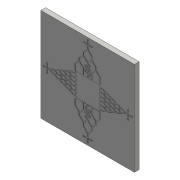
# Autodesk Inventor part: Tree+Mixer
Saved by Autodesk Inventor 2016 (Build 200138000, 138)
## iProperties
Created: 2018-10-05
Part Number: Tree+Mixer
Material: Genérico
Document SubType Name: Modeling
Designer: Joseahpacho
Density: 1 g/cm^3
Appearance: Valor por defecto
Author: Joseahpacho
Autodesk Inventor part; units mm, degrees
ref_plane "YZ Plane" through (0, 0, 0) normal (1, 0, 0) x (0, 1, 0)
ref_plane "XZ Plane" through (0, 0, 0) normal (0, 1, 0) x (-1, 0, 0)
ref_plane "XY Plane" through (0, 0, 0) normal (0, 0, 1) x (1, 0, 0)
sketch "Boceto1" plane through (0, 0, 0) normal (0, 1, 0) x (-1, 0, 0)
  line L0 (29.6771, 58.45) -> (33.6771, 60.45)
  line L1 (23.4615, 55.55) -> (24.4631, 55.55)
  line L2 (24.4631, 55.55) -> (27.5631, 54)
  line L3 (24.4631, 52.45) -> (27.5631, 54)
  line L4 (25.5755, 56) -> (28.6755, 57.55)
  line L5 (25.5755, 56) -> (28.6755, 54.45)
  line L6 (25.5755, 52) -> (28.6755, 50.45)
  line L7 (23.4615, 52.45) -> (24.4631, 52.45)
  line L8 (23.4615, 52.45) -> (24.4631, 52.45)
  line L9 (24.4631, 52.45) -> (23.4615, 52.45)
  line L10 (25.3631, 48) -> (28.4631, 49.55)
  line L11 (24.4631, 51.55) -> (27.4568, 50.0531)
  line L12 (23.4615, 51.55) -> (24.4631, 51.55)
  line L13 (23.4615, 51.55) -> (24.4631, 51.55)
  line L14 (24.2506, 48.45) -> (27.4568, 50.0531)
  line L15 (23.4615, 48.45) -> (24.2506, 48.45)
  line L16 (24.2506, 48.45) -> (23.4615, 48.45)
  line L17 (23.4615, 48.45) -> (24.2506, 48.45)
  line L18 (33.8896, 56.45) -> (35.8375, 56.45)
  line L19 (29.4647, 54.45) -> (32.6709, 56.0531)
  line L20 (33.6771, 52.45) -> (36.0499, 52.45)
  line L21 (33.6771, 51.55) -> (36.0499, 51.55)
  line L22 (29.4647, 53.55) -> (32.5647, 52)
  line L23 (29.4647, 50.45) -> (32.5647, 52)
  line L24 (29.4647, 54.45) -> (28.6755, 54.45)
  line L25 (28.6755, 54.45) -> (29.4647, 54.45)
  line L26 (29.4647, 53.55) -> (28.6755, 53.55)
  line L27 (28.6755, 53.55) -> (29.4647, 53.55)
  line L28 (28.4631, 49.55) -> (29.4647, 49.55)
  line L29 (28.4631, 49.55) -> (29.4647, 49.55)
  line L30 (29.4647, 49.55) -> (28.4631, 49.55)
  line L31 (29.4647, 50.45) -> (28.6755, 50.45)
  line L32 (28.6755, 50.45) -> (29.4647, 50.45)
  line L33 (28.6755, 50.45) -> (29.4647, 50.45)
  line L34 (28.6755, 54.45) -> (29.4647, 54.45)
  line L35 (29.4647, 49.55) -> (32.4585, 48.0531)
  line L36 (30.5771, 50) -> (33.6771, 48.45)
  line L37 (30.5771, 50) -> (33.6771, 51.55)
  line L38 (33.4647, 47.55) -> (36.0499, 47.55)
  line L39 (33.6771, 48.45) -> (36.0499, 48.45)
  line L40 (30.5771, 54) -> (33.6771, 52.45)
  line L41 (30.5771, 54) -> (33.6771, 55.55)
  line L42 (33.6771, 52.45) -> (35.8375, 52.45)
  line L43 (33.6771, 55.55) -> (35.8375, 55.55)
  line L44 (33.6771, 55.55) -> (36.0499, 55.55)
  line L45 (33.8896, 56.45) -> (36.0499, 56.45)
  line L46 (28.6755, 53.55) -> (29.4647, 53.55)
  line L47 (29.2522, 46.45) -> (28.4631, 46.45)
  line L48 (28.4631, 46.45) -> (29.2522, 46.45)
  line L49 (33.4647, 47.55) -> (35.625, 47.55)
  line L50 (28.4631, 46.45) -> (29.2522, 46.45)
  line L51 (28.2506, 45.55) -> (29.2522, 45.55)
  line L52 (28.2506, 45.55) -> (29.2522, 45.55)
  line L53 (33.4647, 44.45) -> (35.625, 44.45)
  line L54 (33.4647, 44.45) -> (36.0499, 44.45)
  line L55 (29.2522, 45.55) -> (32.246, 44.0531)
  line L56 (29.0398, 42.45) -> (32.246, 44.0531)
  line L57 (30.1522, 42) -> (33.2522, 43.55)
  line L58 (33.2522, 40.45) -> (36.0499, 40.45)
  line L59 (33.0398, 39.55) -> (36.0499, 39.55)
  line L60 (30.1522, 42) -> (33.2522, 40.45)
  line L61 (28.2506, 42.45) -> (29.0398, 42.45)
  line L62 (29.0398, 42.45) -> (28.2506, 42.45)
  line L63 (28.0382, 41.55) -> (29.0398, 41.55)
  line L64 (29.0398, 41.55) -> (28.0382, 41.55)
  line L65 (25.1506, 44) -> (28.2506, 42.45)
  line L66 (24.2506, 47.55) -> (27.2444, 46.0531)
  line L67 (15.1474, 48) -> (18.2474, 46.45)
  line L68 (19.0366, 45.55) -> (18.035, 45.55)
  line L69 (20.3615, 54) -> (23.4615, 55.55)
  line L70 (20.3615, 54) -> (23.4615, 52.45)
  line L71 (19.249, 54.45) -> (23.249, 56.45)
  line L72 (19.0366, 46.45) -> (22.2428, 48.0531)
  line L73 (19.249, 53.55) -> (22.349, 52)
  line L74 (19.249, 54.45) -> (18.2474, 54.45)
  line L75 (19.249, 53.55) -> (18.2474, 53.55)
  line L76 (18.2474, 53.55) -> (19.249, 53.55)
  line L77 (18.035, 54.45) -> (19.249, 54.45)
  line L78 (19.249, 50.45) -> (22.349, 52)
  line L79 (24.4631, 55.55) -> (23.4615, 55.55)
  line L80 (20.3615, 50) -> (23.4615, 51.55)
  line L81 (20.3615, 50) -> (23.4615, 48.45)
  line L82 (20.149, 46) -> (23.249, 44.45)
  line L83 (20.149, 46) -> (23.249, 47.55)
  line L84 (19.249, 49.55) -> (22.2428, 48.0531)
  line L85 (19.249, 50.45) -> (18.2474, 50.45)
  line L86 (19.249, 49.55) -> (18.2474, 49.55)
  line L87 (14.035, 52.45) -> (18.035, 54.45)
  line L88 (14.035, 51.55) -> (17.135, 50)
  line L89 (14.035, 47.55) -> (18.035, 45.55)
  line L90 (19.0366, 46.45) -> (18.2474, 46.45)
  line L91 (24.4631, 56.45) -> (23.4615, 56.45)
  line L92 (24.0382, 43.55) -> (23.0366, 43.55)
  line L93 (24.0382, 44.45) -> (23.249, 44.45)
  line L94 (23.249, 47.55) -> (24.2506, 47.55)
  line L95 (23.249, 47.55) -> (24.2506, 47.55)
  line L96 (23.249, 44.45) -> (24.0382, 44.45)
  line L97 (23.0366, 43.55) -> (24.0382, 43.55)
  line L98 (24.2506, 47.55) -> (23.249, 47.55)
  line L99 (24.4631, 51.55) -> (23.4615, 51.55)
  line L100 (25.5755, 52) -> (28.6755, 53.55)
  line L101 (25.3631, 48) -> (28.4631, 46.45)
  line L102 (25.1506, 44) -> (28.2506, 45.55)
  line L103 (29.2522, 45.55) -> (28.2506, 45.55)
  line L104 (24.0382, 43.55) -> (28.0382, 41.55)
  line L105 (30.3647, 46) -> (33.4647, 47.55)
  line L106 (30.3647, 46) -> (33.4647, 44.45)
  line L107 (33.6771, 48.45) -> (35.8375, 48.45)
  line L108 (33.6771, 51.55) -> (35.8375, 51.55)
  line L109 (29.0398, 41.55) -> (33.0398, 39.55)
  line L110 (33.2522, 43.55) -> (36.0499, 43.55)
  line L111 (33.2522, 43.55) -> (36.0499, 43.55)
  line L112 (38.1364, 37.5) -> (45.0192, 37.5)
  line L113 (37.3383, 44.9144) -> (37.3383, 47.0856)
  line L114 (37.3383, 40.9144) -> (37.3383, 43.0856)
  line L115 (36.0499, 48.45) -> (37.3383, 48.9144)
  line L116 (36.0499, 47.55) -> (37.3383, 47.0856)
  line L117 (36.0499, 44.45) -> (37.3383, 44.9144)
  line L118 (36.0499, 43.55) -> (37.3383, 43.0856)
  line L119 (37.3383, 37.9747) -> (37.3383, 39.0856)
  line L120 (36.0499, 40.45) -> (37.3383, 40.9144)
  line L121 (36.0499, 39.55) -> (37.3383, 39.0856)
  line L122 (29.2522, 46.45) -> (32.4585, 48.0531)
  line L123 (24.0382, 44.45) -> (27.2444, 46.0531)
  line L124 (37.0192, 30.9258) -> (37.0192, 36.3828)
  line L125 (37.0192, 36.3828) -> (38.1364, 37.5)
  line L126 (36.1192, 36.7556) -> (37.3383, 37.9747)
  line L127 (36.1192, 30.553) -> (36.1192, 36.7556)
  line L128 (9.0334, 50.45) -> (8.0318, 50.45)
  line L129 (9.0334, 49.55) -> (8.0318, 49.55)
  line L130 (90.805, 49.55) -> (86.805, 47.55)
  line L131 (80.8018, 53.55) -> (81.5909, 53.55)
  line L132 (80.5893, 46.45) -> (81.5909, 46.45)
  line L133 (80.5893, 49.55) -> (81.5909, 49.55)
  line L134 (41.0192, 26.9258) -> (45.0192, 30.9258)
  line L135 (30.7896, 58) -> (33.8896, 59.55)
  line L136 (29.6771, 58.45) -> (28.6755, 58.45)
  line L137 (28.4631, 58.45) -> (29.6771, 58.45)
  line L138 (29.6771, 57.55) -> (28.6755, 57.55)
  line L139 (28.6755, 57.55) -> (29.6771, 57.55)
  line L140 (30.7896, 58) -> (33.8896, 56.45)
  line L141 (29.6771, 57.55) -> (32.6709, 56.0531)
  line L142 (33.6771, 60.45) -> (36.0499, 60.45)
  line L143 (33.8896, 59.55) -> (36.0499, 59.55)
  line L144 (36.0499, 59.55) -> (37.3383, 59.0856)
  line L145 (36.0499, 60.45) -> (37.3383, 60.9144)
  line L146 (37.3383, 56.9144) -> (37.3383, 59.0856)
  line L147 (36.0499, 56.45) -> (37.3383, 56.9144)
  line L148 (36.0499, 55.55) -> (37.3383, 55.0856)
  line L149 (37.3383, 52.9144) -> (37.3383, 55.0856)
  line L150 (36.0499, 52.45) -> (37.3383, 52.9144)
  line L151 (23.249, 56.45) -> (24.4631, 56.45)
  line L152 (36.0499, 51.55) -> (37.3383, 51.0856)
  line L153 (37.3383, 48.9144) -> (37.3383, 51.0856)
  line L154 (80.5893, 50.45) -> (81.5909, 50.45)
  line L155 (51.6187, 35.5068) -> (50.9692, 35.5068)
  line L156 (80.5893, 45.55) -> (81.5909, 45.55)
  line L157 (51.6187, 34.6068) -> (50.8219, 34.6068)
  line L158 (81.8034, 45.55) -> (80.5893, 45.55)
  line L159 (84.6909, 48) -> (81.5909, 46.45)
  line L160 (85.8034, 47.55) -> (81.8034, 45.55)
  line L161 (62.3383, 38.1364) -> (62.3383, 39.0248)
  line L162 (0, 0) -> (0, 100)
  line L163 (0, 100) -> (100, 100)
  line L164 (100, 100) -> (100, 0)
  line L165 (100, 0) -> (0, 0)
  line L166 (37.3383, 60.9144) -> (37.3383, 62.0253)
  line L167 (45.0192, 30.9258) -> (45.0192, 37.5)
  line L168 (45.9192, 30.553) -> (45.9192, 37.5)
  line L169 (84.6909, 52) -> (81.5909, 50.45)
  line L170 (84.6909, 48) -> (81.5909, 49.55)
  line L171 (85.8034, 48.45) -> (82.7034, 50)
  line L172 (24.4631, 56.45) -> (28.4631, 58.45)
  line L173 (49.4692, 37.5) -> (45.9192, 37.5)
  line L174 (85.8034, 47.55) -> (86.805, 47.55)
  line L175 (41.0192, 73.0742) -> (45.0192, 69.0742)
  line L176 (38.1364, 62.5) -> (45.0192, 62.5)
  line L177 (48.2197, 64.4932) -> (48.8692, 64.4932)
  line L178 (48.2197, 65.3932) -> (49.0165, 65.3932)
  line L179 (85.8034, 48.45) -> (86.5925, 48.45)
  line L180 (50.3692, 63.9776) -> (50.3692, 62.5)
  line L181 (84.6909, 52) -> (81.5909, 53.55)
  line L182 (85.8034, 51.55) -> (86.5925, 51.55)
  line L183 (85.8034, 52.45) -> (86.805, 52.45)
  line L184 (80.8018, 54.45) -> (81.8034, 54.45)
  line L185 (74.6877, 56) -> (71.5877, 57.55)
  line L186 (75.8002, 56.45) -> (71.8002, 58.45)
  line L187 (71.3753, 50.45) -> (70.3737, 50.45)
  line L188 (41.4692, 73.897) -> (41.4692, 74.8986)
  line L189 (40.5692, 73.897) -> (40.5692, 74.8986)
  line L190 (74.4753, 52) -> (71.3753, 53.55)
  line L191 (75.5877, 51.55) -> (72.3815, 49.9469)
  line L192 (41.4692, 73.897) -> (45.9192, 69.447)
  line L193 (76.3769, 48.45) -> (75.3753, 48.45)
  line L194 (76.3769, 47.55) -> (75.3753, 47.55)
  line L195 (40.5692, 73.897) -> (36.1192, 69.447)
  line L196 (41.0192, 73.0742) -> (37.0192, 69.0742)
  line L197 (76.3769, 47.55) -> (75.3753, 47.55)
  line L198 (76.3769, 44.45) -> (75.3753, 44.45)
  line L199 (45.0192, 69.0742) -> (45.0192, 62.5)
  line L200 (45.9192, 69.447) -> (45.9192, 62.5)
  line L201 (45.9192, 62.5) -> (49.4692, 62.5)
  line L202 (37.0192, 69.0742) -> (37.0192, 63.6172)
  line L203 (36.1192, 69.447) -> (36.1192, 63.2444)
  line L204 (37.0192, 63.6172) -> (38.1364, 62.5)
  line L205 (36.1192, 63.2444) -> (37.3383, 62.0253)
  line L206 (79.4769, 46) -> (76.3769, 44.45)
  line L207 (80.5893, 45.55) -> (76.5893, 43.55)
  line L208 (53.9192, 69.447) -> (53.9192, 62.5)
  line L209 (58.3692, 73.897) -> (53.9192, 69.447)
  line L210 (63.7884, 48.45) -> (62.5, 48.9144)
  line L211 (63.7884, 55.55) -> (62.5, 55.0856)
  line L212 (59.2692, 74.3978) -> (59.2692, 73.897)
  line L213 (63.7884, 59.55) -> (62.5, 59.0856)
  line L214 (63.7884, 60.45) -> (62.5, 60.9144)
  line L215 (53.9192, 37.5) -> (50.3692, 37.5)
  line L216 (62.5, 59.0856) -> (62.5, 56.9144)
  line L217 (62.5, 55.0856) -> (62.5, 52.9144)
  line L218 (63.7884, 56.45) -> (62.5, 56.9144)
  line L219 (63.7884, 52.45) -> (62.5, 52.9144)
  line L220 (63.7884, 51.55) -> (62.5, 51.0856)
  line L221 (70.3737, 46.45) -> (67.2737, 48)
  line L222 (49.4692, 36.0224) -> (49.4692, 37.5)
  line L223 (70.3737, 45.55) -> (71.1628, 45.55)
  line L224 (50.3692, 62.5) -> (53.9192, 62.5)
  line L225 (71.1628, 46.45) -> (70.3737, 46.45)
  line L226 (66.1612, 51.55) -> (63.7884, 51.55)
  line L227 (63.7192, 63.2444) -> (62.5, 62.0253)
  line L228 (63.7192, 69.447) -> (63.7192, 63.2444)
  line L229 (62.8192, 69.0742) -> (62.8192, 63.6172)
  line L230 (54.8192, 62.5) -> (61.702, 62.5)
  line L231 (59.2692, 73.897) -> (63.7192, 69.447)
  line L232 (58.8192, 73.0742) -> (62.8192, 69.0742)
  line L233 (54.8192, 69.0742) -> (54.8192, 62.5)
  line L234 (58.8192, 73.0742) -> (54.8192, 69.0742)
  line L235 (62.8192, 63.6172) -> (61.702, 62.5)
  line L236 (15.1474, 52) -> (18.2474, 50.45)
  line L237 (14.035, 48.45) -> (17.135, 50)
  line L238 (14.035, 51.55) -> (13.2458, 51.55)
  line L239 (14.035, 52.45) -> (13.0334, 52.45)
  line L240 (71.1628, 45.55) -> (70.3737, 45.55)
  line L241 (71.1628, 46.45) -> (70.3737, 46.45)
  line L242 (71.1628, 49.55) -> (70.3737, 49.55)
  line L243 (71.1628, 49.55) -> (70.3737, 49.55)
  line L244 (71.1628, 45.55) -> (70.3737, 45.55)
  line L245 (71.5877, 57.55) -> (70.7986, 57.55)
  line L246 (71.8002, 58.45) -> (70.7986, 58.45)
  line L247 (71.3753, 50.45) -> (70.3737, 50.45)
  line L248 (71.3753, 53.55) -> (70.5861, 53.55)
  line L249 (14.035, 48.45) -> (13.2458, 48.45)
  line L250 (15.1474, 48) -> (18.2474, 49.55)
  line L251 (14.035, 47.55) -> (13.0334, 47.55)
  line L252 (10.1458, 50) -> (13.2458, 51.55)
  line L253 (10.1458, 50) -> (13.2458, 48.45)
  line L254 (9.0334, 49.55) -> (13.0334, 47.55)
  line L255 (9.0334, 50.45) -> (13.0334, 52.45)
  line L256 (15.1474, 52) -> (18.2474, 53.55)
  line L257 (71.3753, 53.55) -> (70.5861, 53.55)
  line L258 (71.5877, 54.45) -> (70.5861, 54.45)
  line L259 (71.5877, 54.45) -> (70.5861, 54.45)
  line L260 (58.3692, 74.3978) -> (58.3692, 73.897)
  line L261 (49.4692, 89.045) -> (49.4692, 90.0466)
  line L262 (74.2628, 48) -> (71.1628, 49.55)
  line L263 (74.2628, 48) -> (71.1628, 46.45)
  line L264 (74.4753, 52) -> (71.3753, 50.45)
  line L265 (74.6877, 56) -> (71.5877, 54.45)
  line L266 (75.8002, 55.55) -> (72.594, 53.9469)
  line L267 (75.5877, 52.45) -> (72.594, 53.9469)
  line L268 (75.3753, 47.55) -> (72.2753, 46)
  line L269 (76.5893, 43.55) -> (75.3753, 43.55)
  line L270 (75.3753, 47.55) -> (76.3769, 47.55)
  line L271 (76.3769, 48.45) -> (75.3753, 48.45)
  line L272 (75.3753, 48.45) -> (76.3769, 48.45)
  line L273 (75.3753, 48.45) -> (72.3815, 49.9469)
  line L274 (50.3692, 76.3978) -> (50.3692, 76.025)
  line L275 (50.3692, 89.045) -> (50.3692, 90.0466)
  line L276 (49.4692, 89.045) -> (45.0192, 84.595)
  line L277 (49.9192, 88.2222) -> (45.9192, 84.2222)
  line L278 (50.3692, 89.045) -> (54.8192, 84.595)
  line L279 (49.9192, 88.2222) -> (53.9192, 84.2222)
  line L280 (45.0192, 84.595) -> (45.0192, 82.2222)
  line L281 (45.9192, 84.2222) -> (45.9192, 82.2222)
  line L282 (45.9192, 81.2206) -> (45.9192, 82.2222)
  line L283 (45.0192, 81.2206) -> (45.0192, 82.2222)
  line L284 (53.9192, 84.2222) -> (53.9192, 82.2222)
  line L285 (54.8192, 84.595) -> (54.8192, 82.2222)
  line L286 (53.9192, 81.2206) -> (53.9192, 82.2222)
  line L287 (54.8192, 81.2206) -> (54.8192, 82.2222)
  line L288 (53.9192, 81.2206) -> (49.9192, 77.2206)
  line L289 (54.3692, 80.3978) -> (50.3692, 76.3978)
  line L290 (54.3692, 80.3978) -> (58.3692, 76.3978)
  line L291 (54.8192, 81.2206) -> (59.2692, 76.7706)
  line L292 (59.2692, 76.7706) -> (59.2692, 74.3978)
  line L293 (58.3692, 76.3978) -> (58.3692, 74.3978)
  line L294 (45.4692, 80.3978) -> (49.4692, 76.3978)
  line L295 (45.4692, 80.3978) -> (41.4692, 76.3978)
  line L296 (45.0192, 81.2206) -> (40.5692, 76.7706)
  line L297 (40.5692, 76.7706) -> (40.5692, 74.3978)
  line L298 (41.4692, 76.3978) -> (41.4692, 74.3978)
  line L299 (45.9192, 81.2206) -> (49.9192, 77.2206)
  line L300 (19.0366, 45.55) -> (23.0366, 43.55)
  line L301 (61.702, 37.5) -> (54.8192, 37.5)
  line L302 (54.8192, 30.9258) -> (54.8192, 37.5)
  line L303 (40.5692, 26.103) -> (36.1192, 30.553)
  line L304 (63.7192, 36.7556) -> (62.3383, 38.1364)
  line L305 (62.8192, 36.3828) -> (61.702, 37.5)
  line L306 (62.8192, 30.9258) -> (62.8192, 36.3828)
  line L307 (53.9192, 30.553) -> (53.9192, 37.5)
  line L308 (63.7192, 30.553) -> (63.7192, 36.7556)
  line L309 (58.8192, 26.9258) -> (54.8192, 30.9258)
  line L310 (58.8192, 26.9258) -> (62.8192, 30.9258)
  line L311 (58.3692, 26.103) -> (58.3692, 25.1014)
  line L312 (40.5692, 23.2294) -> (40.5692, 25.6022)
  line L313 (45.4692, 19.6022) -> (41.4692, 23.6022)
  line L314 (45.9192, 18.7794) -> (49.9192, 22.7794)
  line L315 (59.2692, 26.103) -> (63.7192, 30.553)
  line L316 (41.0192, 26.9258) -> (37.0192, 30.9258)
  line L317 (58.3692, 26.103) -> (53.9192, 30.553)
  line L318 (59.2692, 26.103) -> (59.2692, 25.1014)
  line L319 (49.4692, 23.6022) -> (49.4692, 23.975)
  line L320 (40.5692, 25.6022) -> (40.5692, 26.103)
  line L321 (41.4692, 25.6022) -> (41.4692, 26.103)
  line L322 (41.4692, 26.103) -> (45.9192, 30.553)
  line L323 (41.4692, 23.6022) -> (41.4692, 25.6022)
  line L324 (53.9192, 18.7794) -> (49.9192, 22.7794)
  line L325 (45.0192, 18.7794) -> (40.5692, 23.2294)
  line L326 (62.5, 51.0856) -> (62.5, 48.9144)
  line L327 (70.7986, 57.55) -> (67.5924, 55.9469)
  line L328 (70.3737, 50.45) -> (71.3753, 50.45)
  line L329 (66.1612, 48.45) -> (63.7884, 48.45)
  line L330 (66.1612, 47.55) -> (63.7884, 47.55)
  line L331 (66.1612, 51.55) -> (64.0009, 51.55)
  line L332 (66.1612, 48.45) -> (64.0009, 48.45)
  line L333 (66.1612, 47.55) -> (64.0009, 47.55)
  line L334 (66.3737, 52.45) -> (63.7884, 52.45)
  line L335 (66.3737, 55.55) -> (63.7884, 55.55)
  line L336 (66.3737, 52.45) -> (64.2133, 52.45)
  line L337 (66.3737, 55.55) -> (64.2133, 55.55)
  line L338 (66.5861, 56.45) -> (63.7884, 56.45)
  line L339 (66.5861, 56.45) -> (63.7884, 56.45)
  line L340 (69.2612, 50) -> (66.1612, 51.55)
  line L341 (69.2612, 50) -> (66.1612, 48.45)
  line L342 (69.6861, 58) -> (66.5861, 59.55)
  line L343 (69.4737, 54) -> (66.3737, 52.45)
  line L344 (69.4737, 54) -> (66.3737, 55.55)
  line L345 (70.3737, 49.55) -> (67.2737, 48)
  line L346 (70.3737, 50.45) -> (67.3799, 51.9469)
  line L347 (70.7986, 57.55) -> (71.5877, 57.55)
  line L348 (70.7986, 58.45) -> (71.8002, 58.45)
  line L349 (71.1628, 42.45) -> (70.1612, 42.45)
  line L350 (70.3737, 46.45) -> (71.1628, 46.45)
  line L351 (70.3737, 49.55) -> (71.1628, 49.55)
  line L352 (70.5861, 54.45) -> (71.5877, 54.45)
  line L353 (74.2628, 44) -> (71.1628, 42.45)
  line L354 (74.2628, 44) -> (71.1628, 45.55)
  line L355 (75.3753, 44.45) -> (72.2753, 46)
  line L356 (75.3753, 44.45) -> (76.3769, 44.45)
  line L357 (70.5861, 53.55) -> (71.3753, 53.55)
  line L358 (70.1612, 42.45) -> (67.1674, 43.9469)
  line L359 (65.9487, 40.45) -> (63.7884, 40.45)
  line L360 (63.7884, 39.55) -> (62.3383, 39.0248)
  line L361 (70.1612, 41.55) -> (71.1628, 41.55)
  line L362 (69.0487, 42) -> (65.9487, 40.45)
  line L363 (70.3737, 45.55) -> (67.1674, 43.9469)
  line L364 (63.7884, 44.45) -> (62.5, 44.9144)
  line L365 (70.1612, 41.55) -> (66.1612, 39.55)
  line L366 (59.2692, 23.2294) -> (59.2692, 25.6022)
  line L367 (58.3692, 23.6022) -> (58.3692, 25.6022)
  line L368 (54.3692, 19.6022) -> (58.3692, 23.6022)
  line L369 (54.8192, 18.7794) -> (59.2692, 23.2294)
  line L370 (54.8192, 18.7794) -> (54.8192, 17.7778)
  line L371 (53.9192, 18.7794) -> (53.9192, 17.7778)
  line L372 (54.3692, 19.6022) -> (50.3692, 23.6022)
  line L373 (54.8192, 15.405) -> (54.8192, 17.7778)
  line L374 (53.9192, 15.7778) -> (53.9192, 17.7778)
  line L375 (45.4692, 19.6022) -> (49.4692, 23.6022)
  line L376 (45.9192, 18.7794) -> (45.9192, 17.7778)
  line L377 (45.0192, 18.7794) -> (45.0192, 17.7778)
  line L378 (45.9192, 15.7778) -> (45.9192, 17.7778)
  line L379 (45.0192, 15.405) -> (45.0192, 17.7778)
  line L380 (50.3692, 10.955) -> (54.8192, 15.405)
  line L381 (49.4692, 10.955) -> (49.4692, 9.9534)
  line L382 (49.9192, 11.7778) -> (45.9192, 15.7778)
  line L383 (49.4692, 10.955) -> (45.0192, 15.405)
  line L384 (50.3692, 10.955) -> (50.3692, 9.9534)
  line L385 (49.9192, 11.7778) -> (53.9192, 15.7778)
  line L386 (66.1612, 39.55) -> (63.7884, 39.55)
  line L387 (63.7884, 40.45) -> (62.5, 40.9144)
  line L388 (62.5, 43.0856) -> (62.5, 40.9144)
  line L389 (63.7884, 43.55) -> (62.5, 43.0856)
  line L390 (65.9487, 43.55) -> (64.0009, 43.55)
  line L391 (65.9487, 43.55) -> (63.7884, 43.55)
  line L392 (66.1612, 44.45) -> (63.7884, 44.45)
  line L393 (62.5, 47.0856) -> (62.5, 44.9144)
  line L394 (69.0487, 42) -> (65.9487, 43.55)
  line L395 (70.1612, 42.45) -> (71.1628, 42.45)
  line L396 (63.7884, 47.55) -> (62.5, 47.0856)
  line L397 (69.2612, 46) -> (66.1612, 44.45)
  line L398 (69.2612, 46) -> (66.1612, 47.55)
  line L399 (66.1612, 44.45) -> (64.0009, 44.45)
  line L400 (70.7986, 58.45) -> (66.7986, 60.45)
  line L401 (66.5861, 59.55) -> (63.7884, 59.55)
  line L402 (66.7986, 60.45) -> (63.7884, 60.45)
  line L403 (69.6861, 58) -> (66.5861, 56.45)
  line L404 (70.5861, 54.45) -> (67.5924, 55.9469)
  line L405 (70.5861, 53.55) -> (67.3799, 51.9469)
  line L406 (71.3753, 41.55) -> (70.1612, 41.55)
  line L407 (75.3753, 43.55) -> (76.3769, 43.55)
  line L408 (75.3753, 43.55) -> (71.3753, 41.55)
  line L409 (62.5, 62.0253) -> (62.5, 60.9144)
  line L410 (75.5877, 51.55) -> (76.3769, 51.55)
  line L411 (75.5877, 52.45) -> (76.5893, 52.45)
  line L412 (75.8002, 55.55) -> (76.5893, 55.55)
  line L413 (75.8002, 56.45) -> (76.8018, 56.45)
  line L414 (80.5893, 50.45) -> (77.5956, 51.9469)
  line L415 (80.8018, 53.55) -> (77.5956, 51.9469)
  line L416 (79.6893, 54) -> (76.5893, 52.45)
  line L417 (79.6893, 54) -> (76.5893, 55.55)
  line L418 (80.8018, 54.45) -> (76.8018, 56.45)
  line L419 (76.5893, 55.55) -> (75.8002, 55.55)
  line L420 (76.8018, 56.45) -> (75.8002, 56.45)
  line L421 (76.5893, 52.45) -> (75.5877, 52.45)
  line L422 (76.5893, 52.45) -> (75.5877, 52.45)
  line L423 (76.3769, 51.55) -> (75.5877, 51.55)
  line L424 (76.3769, 51.55) -> (75.5877, 51.55)
  line L425 (79.4769, 50) -> (76.3769, 51.55)
  line L426 (80.5893, 49.55) -> (77.4893, 48)
  line L427 (79.4769, 50) -> (76.3769, 48.45)
  line L428 (79.4769, 46) -> (76.3769, 47.55)
  line L429 (80.5893, 46.45) -> (77.4893, 48)
  line L430 (85.8034, 52.45) -> (81.8034, 54.45)
  line L431 (81.5909, 46.45) -> (80.5893, 46.45)
  line L432 (85.8034, 51.55) -> (82.7034, 50)
  line L433 (90.805, 50.45) -> (91.8066, 50.45)
  line L434 (90.805, 50.45) -> (86.805, 52.45)
  line L435 (89.6925, 50) -> (86.5925, 51.55)
  line L436 (89.6925, 50) -> (86.5925, 48.45)
  line L437 (90.805, 49.55) -> (91.8066, 49.55)
  line L438 (8.0318, 49.55) -> (7.0772, 48.5954)
  line L439 (7.0772, 48.5954) -> (7.0772, 46.207)
  line L440 (6.1772, 46.207) -> (6.1772, 48.9682)
  arc A0 (6.1772, 46.207) -> (7.0772, 46.207) centre (6.6272, 45.607) ccw
  arc A1 (50.3692, 36.1068) -> (50.9692, 35.5068) centre (50.9692, 36.1068) ccw
  arc A2 (49.4692, 36.1068) -> (50.9692, 34.6068) centre (50.9692, 36.1068) ccw
  line L441 (48.2197, 33.4068) -> (51.6187, 33.4068)
  arc A3 (51.6187, 32.5068) -> (51.6187, 35.5068) centre (51.6187, 34.0068) ccw
  line L442 (48.2197, 31.3068) -> (51.6187, 31.3068)
  arc A4 (48.2197, 33.4068) -> (48.2197, 30.4068) centre (48.2197, 31.9068) ccw
  arc A5 (48.2197, 32.5068) -> (48.2197, 31.3068) centre (48.2197, 31.9068) ccw
  line L443 (51.6187, 32.5068) -> (48.2197, 32.5068)
  line L444 (50.3692, 37.5) -> (50.3692, 36.1068)
  line L445 (49.4692, 62.5) -> (49.4692, 63.8932)
  line L446 (51.6187, 70.7932) -> (48.2197, 70.7932)
  arc A6 (48.2197, 70.7932) -> (48.2197, 69.5932) centre (48.2197, 70.1932) ccw
  line L447 (48.2197, 69.5932) -> (51.6187, 69.5932)
  line L448 (51.6187, 66.5932) -> (48.2197, 66.5932)
  arc A7 (48.2197, 66.5932) -> (48.2197, 65.3932) centre (48.2197, 65.9932) ccw
  line L449 (48.2197, 71.6932) -> (51.6187, 71.6932)
  line L450 (51.6187, 72.8932) -> (48.2197, 72.8932)
  line L451 (51.6187, 68.6932) -> (48.2197, 68.6932)
  arc A8 (48.2197, 71.6932) -> (48.2197, 68.6932) centre (48.2197, 70.1932) ccw
  arc A9 (51.6187, 67.4932) -> (51.6187, 68.6932) centre (51.6187, 68.0932) ccw
  line L452 (48.2197, 67.4932) -> (51.6187, 67.4932)
  arc A10 (48.2197, 67.4932) -> (48.2197, 64.4932) centre (48.2197, 65.9932) ccw
  arc A11 (49.4692, 63.8932) -> (48.8692, 64.4932) centre (48.8692, 63.8932) ccw
  arc A12 (50.3692, 63.8932) -> (48.8692, 65.3932) centre (48.8692, 63.8932) ccw
  arc A13 (51.6187, 66.5932) -> (51.6187, 69.5932) centre (51.6187, 68.0932) ccw
  arc A14 (51.6187, 70.7932) -> (51.6187, 73.7932) centre (51.6187, 72.2932) ccw
  line L453 (7.0772, 53.793) -> (7.0772, 51.4046)
  line L454 (6.1772, 51.0318) -> (6.1772, 53.793)
  arc A15 (7.0772, 53.793) -> (6.1772, 53.793) centre (6.6272, 54.393) ccw
  line L455 (7.0772, 51.4046) -> (8.0318, 50.45)
  line L456 (6.1772, 48.9682) -> (6.759, 49.55)
  line L457 (6.759, 50.45) -> (6.1772, 51.0318)
  line L458 (6.759, 49.55) -> (3.402, 49.55)
  line L459 (3.402, 50.45) -> (6.759, 50.45)
  arc A16 (3.402, 50.45) -> (3.402, 49.55) centre (2.802, 50) ccw
  line L460 (48.9646, 75.8932) -> (49.4692, 76.3978)
  arc A17 (48.2197, 74.9932) -> (48.2197, 73.7932) centre (48.2197, 74.3932) ccw
  line L461 (48.2197, 73.7932) -> (51.6187, 73.7932)
  line L462 (49.4692, 90.0466) -> (49.4692, 92.0466)
  line L463 (49.4692, 92.0466) -> (48.5146, 93.0012)
  line L464 (48.5146, 93.0012) -> (46.1262, 93.0012)
  arc A18 (46.1262, 93.9012) -> (46.1262, 93.0012) centre (45.5262, 93.4512) ccw
  line L465 (46.1262, 93.9012) -> (48.8874, 93.9012)
  line L466 (48.8874, 93.9012) -> (49.4692, 93.3194)
  line L467 (49.4692, 93.3194) -> (49.4692, 96.6764)
  arc A19 (50.3692, 96.6764) -> (49.4692, 96.6764) centre (49.9192, 97.2764) ccw
  line L468 (50.3692, 96.6764) -> (50.3692, 93.3194)
  line L469 (50.3692, 93.3194) -> (50.951, 93.9012)
  line L470 (50.951, 93.9012) -> (53.7122, 93.9012)
  line L471 (48.5146, 6.9988) -> (49.4692, 7.9534)
  line L472 (49.4692, 7.9534) -> (49.4692, 9.9534)
  line L473 (50.501, 25.0068) -> (51.6187, 25.0068)
  line L474 (51.6187, 24.1068) -> (50.8738, 24.1068)
  arc A20 (51.6187, 24.1068) -> (51.6187, 27.1068) centre (51.6187, 25.6068) ccw
  line L475 (49.4692, 23.975) -> (50.501, 25.0068)
  line L476 (50.8738, 24.1068) -> (50.3692, 23.6022)
  line L477 (48.2197, 75.8932) -> (48.9646, 75.8932)
  arc A21 (48.2197, 75.8932) -> (48.2197, 72.8932) centre (48.2197, 74.3932) ccw
  line L478 (50.3692, 76.025) -> (49.3374, 74.9932)
  line L479 (50.3692, 92.0466) -> (50.3692, 90.0466)
  arc A22 (51.6187, 71.6932) -> (51.6187, 72.8932) centre (51.6187, 72.2932) ccw
  line L480 (53.7122, 93.0012) -> (51.3238, 93.0012)
  arc A23 (51.6187, 28.3068) -> (51.6187, 31.3068) centre (51.6187, 29.8068) ccw
  line L481 (48.2197, 27.1068) -> (51.6187, 27.1068)
  arc A24 (48.2197, 28.3068) -> (48.2197, 27.1068) centre (48.2197, 27.7068) ccw
  arc A25 (48.2197, 29.2068) -> (48.2197, 26.2068) centre (48.2197, 27.7068) ccw
  line L482 (48.2197, 29.2068) -> (51.6187, 29.2068)
  arc A26 (51.6187, 29.2068) -> (51.6187, 30.4068) centre (51.6187, 29.8068) ccw
  line L483 (51.6187, 30.4068) -> (48.2197, 30.4068)
  line L484 (51.6187, 28.3068) -> (48.2197, 28.3068)
  arc A27 (51.6187, 25.0068) -> (51.6187, 26.2068) centre (51.6187, 25.6068) ccw
  line L485 (51.3238, 93.0012) -> (50.3692, 92.0466)
  arc A28 (51.6187, 33.4068) -> (51.6187, 34.6068) centre (51.6187, 34.0068) ccw
  line L486 (51.6187, 26.2068) -> (48.2197, 26.2068)
  line L487 (49.3374, 74.9932) -> (48.2197, 74.9932)
  line L488 (50.3692, 9.9534) -> (50.3692, 7.9534)
  line L489 (50.3692, 7.9534) -> (51.3238, 6.9988)
  line L490 (51.3238, 6.9988) -> (53.7122, 6.9988)
  arc A29 (53.7122, 6.0988) -> (53.7122, 6.9988) centre (54.3122, 6.5488) ccw
  line L491 (53.7122, 6.0988) -> (50.951, 6.0988)
  line L492 (50.951, 6.0988) -> (50.3692, 6.6806)
  line L493 (50.3692, 6.6806) -> (50.3692, 3.3236)
  line L494 (92.7612, 51.4046) -> (92.7612, 53.793)
  line L495 (91.8066, 50.45) -> (92.7612, 51.4046)
  line L496 (93.6612, 53.793) -> (93.6612, 51.0318)
  arc A30 (53.7122, 93.0012) -> (53.7122, 93.9012) centre (54.3122, 93.4512) ccw
  arc A31 (49.4692, 3.3236) -> (50.3692, 3.3236) centre (49.9192, 2.7236) ccw
  line L497 (49.4692, 3.3236) -> (49.4692, 6.6806)
  arc A32 (93.6612, 53.793) -> (92.7612, 53.793) centre (93.2112, 54.393) ccw
  line L498 (49.4692, 6.6806) -> (48.8874, 6.0988)
  line L499 (93.0794, 49.55) -> (93.6612, 48.9682)
  line L500 (48.8874, 6.0988) -> (46.1262, 6.0988)
  line L501 (93.6612, 48.9682) -> (93.6612, 46.207)
  line L502 (92.7612, 46.207) -> (92.7612, 48.5954)
  arc A33 (46.1262, 6.9988) -> (46.1262, 6.0988) centre (45.5262, 6.5488) ccw
  arc A34 (92.7612, 46.207) -> (93.6612, 46.207) centre (93.2112, 45.607) ccw
  line L503 (46.1262, 6.9988) -> (48.5146, 6.9988)
  line L504 (96.4364, 49.55) -> (93.0794, 49.55)
  line L505 (93.0794, 50.45) -> (96.4364, 50.45)
  arc A35 (96.4364, 49.55) -> (96.4364, 50.45) centre (97.0364, 50) ccw
  line L506 (93.6612, 51.0318) -> (93.0794, 50.45)
  line L507 (92.7612, 48.5954) -> (91.8066, 49.55)
  line L508 (100, 100) -> (0, 100)
  line L509 (0, 100) -> (0, 0)
  line L510 (0, 0) -> (100, 0)
  line L511 (100, 0) -> (100, 100)
  constraints: 1024 end point, 72 point on circle, 36 centre point, 28 point on line, 4 midpoint, 2 parallel, 1 horizontal, 1 perpendicular
sketch "Boceto2" plane through (0, 0, 0) normal (0, 1, 0) x (-1, 0, 0)
  line L0 (100, 0) -> (0, 0)
  line L1 (0, 0) -> (0, 100)
  line L2 (0, 100) -> (100, 100)
  line L3 (100, 100) -> (100, 0)
  constraints: 8 end point, 2 parallel, 1 horizontal, 1 perpendicular
extrude "Extrusión1" add sketch "Boceto2" along normal blind 5
extrude "Extrusión2" cut sketch "Boceto1" along normal blind 0.2 contours L0 L142 L145 L166 L205 L203 L195 L189 L297 L296 L283 L280 L276 L261 L462 L463 L464 A18 L465 L466 L467 A19 L468 L469 L470 A30 L480 L485 L479 L275 L278 L285 L287 L291 L292 L212 L231 L228 L227 L409 L214 L402 L400 L246 L186 L413 L418 L184 L430 L183 L434 L433 L495 L494 A32 L496 L506 L505 A35 L504 L499 L501 A34 L502 L507 L437 L130 L174 L160 L158 L156 L207 L269 L408 L406 L361 L365 L386 L360 L161 L304 L308 L315 L318 L366 L369 L370 L373 L380 L384 L488 L489 L490 A29 L491 L492 L493 A31 L497 L498 L500 A33 L503 L471 L472 L381 L383 L379 L377 L325 L312 L320 L303 L127 L126 L119 L121 L59 L109 L63 L104 L92 L300 L68 L89 L251 L254 L129 L438 L439 A0 L440 L456 L458 A16 L459 L457 L454 A15 L453 L455 L128 L255 L239 L87 L77 L74 L71 L151 L91 L172 L137 L136
sketch "Boceto3" plane through (0, 0.2, 0) normal (0, -1, 0) x (1, 0, 0)
  arc A0 (-6.1772, 53.793) -> (-7.0772, 53.793) centre (-6.6272, 54.393) ccw projected
  arc A1 (-3.402, 49.55) -> (-3.402, 50.45) centre (-2.802, 50) ccw projected
  arc A2 (-7.0772, 46.207) -> (-6.1772, 46.207) centre (-6.6272, 45.607) ccw projected
  arc A3 (-46.1262, 6.0988) -> (-46.1262, 6.9988) centre (-45.5262, 6.5488) ccw projected
  arc A4 (-50.3692, 3.3236) -> (-49.4692, 3.3236) centre (-49.9192, 2.7236) ccw projected
  arc A5 (-53.7122, 6.9988) -> (-53.7122, 6.0988) centre (-54.3122, 6.5488) ccw projected
  arc A6 (-93.6612, 46.207) -> (-92.7612, 46.207) centre (-93.2112, 45.607) ccw projected
  arc A7 (-96.4364, 50.45) -> (-96.4364, 49.55) centre (-97.0364, 50) ccw projected
  arc A8 (-92.7612, 53.793) -> (-93.6612, 53.793) centre (-93.2112, 54.393) ccw projected
  arc A9 (-53.7122, 93.9012) -> (-53.7122, 93.0012) centre (-54.3122, 93.4512) ccw projected
  arc A10 (-49.4692, 96.6764) -> (-50.3692, 96.6764) centre (-49.9192, 97.2764) ccw projected
  arc A11 (-46.1262, 93.0012) -> (-46.1262, 93.9012) centre (-45.5262, 93.4512) ccw projected
  circle A12 centre (-6.6272, 54.393) radius 0.35
  circle A13 centre (-2.802, 50) radius 0.35
  circle A14 centre (-6.6272, 45.607) radius 0.35
  circle A15 centre (-45.5262, 6.5488) radius 0.35
  circle A16 centre (-49.9192, 2.7236) radius 0.35
  circle A17 centre (-54.3122, 6.5488) radius 0.35
  circle A18 centre (-93.2112, 45.607) radius 0.35
  circle A19 centre (-97.0364, 50) radius 0.35
  circle A20 centre (-93.2112, 54.393) radius 0.35
  circle A21 centre (-54.3122, 93.4512) radius 0.35
  circle A22 centre (-49.9192, 97.2764) radius 0.35
  circle A23 centre (-45.5262, 93.4512) radius 0.35
  point P0 (0, 0)
  dimension "d4" = 0.7
  dimension "d5" = 0.7
  dimension "d6" = 0.7
  dimension "d7" = 0.7
  dimension "d8" = 0.7
  dimension "d9" = 0.7
  dimension "d10" = 0.7
  dimension "d11" = 0.7
  dimension "d12" = 0.7
  dimension "d13" = 0.7
  dimension "d14" = 0.7
  dimension "d15" = 0.7
  constraints: 12 centre point, 1 coincident
  measures "d4" diameter of A12
  measures "d5" diameter of A13
  measures "d6" diameter of A14
  measures "d7" diameter of A15
  measures "d8" diameter of A16
  measures "d9" diameter of A17
  measures "d10" diameter of A18
  measures "d11" diameter of A19
  measures "d12" diameter of A20
  measures "d13" diameter of A21
  measures "d14" diameter of A22
  measures "d15" diameter of A23
extrude "Extrusión3" cut sketch "Boceto3" against normal through all
